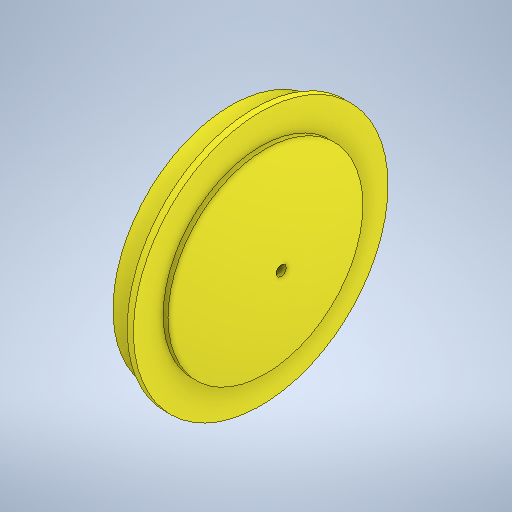
# Autodesk Inventor part: 130 part 2
Saved by Autodesk Inventor 2025.1 (Build 291241000, 241)
## iProperties
Created: 2024-08-01
Part Number: 130 part 2
Material: Aluminum 6061-AHC
Document SubType Name: Modeling
Designer: ffogue
Density: 2.7 g/cm^3
Appearance: Canary
Author: ffogue
Autodesk Inventor part; units mm, degrees
ref_plane "YZ Plane" through (0, 0, 0) normal (1, 0, 0) x (0, 1, 0)
ref_plane "XZ Plane" through (0, 0, 0) normal (0, 1, 0) x (-1, 0, 0)
ref_plane "XY Plane" through (0, 0, 0) normal (0, 0, 1) x (1, 0, 0)
sketch "Sketch1" plane through (0, 0, 0) normal (0, 0, 1) x (1, 0, 0)
  line L0 (0, 0) -> (0, 37.5)
  line L1 (0, 37.5) -> (7.5, 37.5)
  line L2 (7.5, 37.5) -> (7.5, 40.5)
  line L3 (7.5, 40.5) -> (9.5, 40.5)
  line L4 (9.5, 40.5) -> (9.5, 31)
  line L5 (151.3726, 0) -> (0, 0)
  line L6 (9.5, 31) -> (11, 31)
  arc A0 (16, 0) -> (11, 31) centre (-75.9938, 1.0655) ccw
  line L7 (0, 34) -> (9.5, 34) construction
  dimension "d1" = 2
  dimension "d2" = 7.5
  dimension "d4" = 75
  dimension "d5" = 81
  dimension "d6" = 1.5
  dimension "d7" = 92
  dimension "d8" = 68
  dimension "d9" = 16
  dimension "d10" = 62
  constraints: 16 end point, 5 perpendicular, 3 point on line, 2 horizontal, 2 point on circle, 1 centre point, 1 vertical
  measures "d1" distance of L2.end L3.end
  measures "d2" distance of L0.end L1.end
  measures "d4" diameter of L1 L5
  measures "d5" diameter of L3 L5
  measures "d6" distance of L4.end L6.end
  measures "d7" radius of A0
  measures "d8" diameter of L7 L5
  measures "d9" distance from line of A0.start L0
  measures "d10" diameter of L6 L5
revolve "Revolution1" add sketch "Sketch1" angle 360 about axis through (151.3726, 0, 0) along (-1, 0, 0)
sketch "Sketch2" plane through (0, 0, 0) normal (-1, 0, 0) x (0, 0, 1)
  circle A0 centre (0, 0) radius 37.5 projected
  constraints: 1 coincident
hole "Hole1" at (0, 0, 0) direction (1, 0, 0) diameter 68 depth 5.5
sketch "Sketch3" plane through (5.5, 0, 0) normal (-1, 0, 0) x (0, 0, 1)
  circle A0 centre (0, 0) radius 31 projected
  constraints: 1 coincident
hole "Hole2" at (5.5, 0, 0) direction (1, 0, 0) diameter 3.242 end through all thread size "M4x0.7" class "6H" standard "ISO Metric profile"
body "Solid1"
